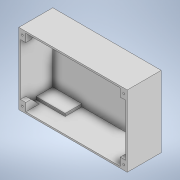
# Autodesk Inventor part: Box2
Saved by Autodesk Inventor 2022 (Build 260153000, 153)
## iProperties
Created: 2021-07-04
Part Number: Box2
Material: Generic
Document SubType Name: Modeling
Designer: Matthijs
Density: 1 g/cm^3
Appearance: Default
Author: Matthijs
Autodesk Inventor part; units mm, degrees
ref_plane "YZ Plane" through (0, 0, 0) normal (1, 0, 0) x (0, 1, 0)
ref_plane "XZ Plane" through (0, 0, 0) normal (0, 1, 0) x (-1, 0, 0)
ref_plane "XY Plane" through (0, 0, 0) normal (0, 0, 1) x (1, 0, 0)
sketch "Sketch7" plane through (0, 0, 0) normal (0, 0, 1) x (1, 0, 0)
  line L0 (100.625, -66.125) -> (-100.625, -66.125)
  line L1 (-100.625, -66.125) -> (-100.625, 66.125)
  line L2 (-100.625, 66.125) -> (100.625, 66.125)
  line L3 (100.625, 66.125) -> (100.625, -66.125)
  line L4 (100.625, -66.125) -> (-100.625, 66.125) construction
  line L5 (-100.625, -66.125) -> (100.625, 66.125) construction
  point P0 (0, 0)
  dimension "d15" = 201.25
  dimension "d16" = 132.25
  constraints: 12 end point, 2 midpoint, 2 parallel, 1 horizontal, 1 perpendicular
  measures "d15" distance of L1.end L2.end
  measures "d16" distance of L0.end L1.end
extrude "Box Outside" add sketch "Sketch7" along normal blind 63
sketch "Sketch8" plane through (0, 0, 63) normal (0, 0, 1) x (1, 0, 0)
  line L0 (-97.625, 63.125) -> (97.625, 63.125)
  line L1 (97.625, 63.125) -> (97.625, -63.125)
  line L2 (97.625, -63.125) -> (-97.625, -63.125)
  line L3 (-97.625, -63.125) -> (-97.625, 63.125)
  line L4 (100.625, 66.125) -> (-100.625, 66.125) projected
  line L5 (-100.625, 66.125) -> (-100.625, -66.125) projected
  line L6 (-100.625, -66.125) -> (100.625, -66.125) projected
  line L7 (100.625, -66.125) -> (100.625, 66.125) projected
  point P0 (0, 0)
  dimension "d19" = 3
  dimension "d20" = 3
  dimension "d21" = 3
  dimension "d22" = 3
  constraints: 8 end point, 2 parallel, 1 horizontal, 1 perpendicular
  measures "d19" distance between parallel lines of L4 L0
  measures "d20" distance between parallel lines of L5 L3
  measures "d21" distance between parallel lines of L6 L2
  measures "d22" distance between parallel lines of L7 L1
extrude "Box Cut" cut sketch "Sketch8" against normal blind 60 contours L0 L1 L2 L3
sketch "Sketch9" plane through (-97.625, -63.125, 63) normal (0, 1, 0) x (1, 0, 0)
  line L0 (0, 0) -> (10, 0)
  line L1 (10, 0) -> (10, 25)
  line L2 (10, 25) -> (0, 25)
  line L3 (0, 25) -> (0, 0)
  point P0 (97.625, 63)
  dimension "d25" = 10
  dimension "d26" = 25
  constraints: 8 end point, 2 parallel, 1 horizontal, 1 perpendicular
  measures "d25" distance of L2.end L1.end
  measures "d26" distance of L1.end L0.end
extrude "ScrewHole Box LB" add sketch "Sketch9" along normal blind 15
sketch "Sketch10" plane through (-97.625, -63.125, 3) normal (0, 1, 0) x (1, 0, 0)
  line L0 (195.25, -60) -> (195.25, 0) projected
  line L1 (195.25, -60) -> (185.25, -60)
  line L2 (185.25, -60) -> (185.25, -35)
  line L3 (185.25, -35) -> (195.25, -35)
  line L4 (195.25, -35) -> (195.25, -60)
  point P0 (97.625, 3)
  dimension "d29" = 10
  dimension "d30" = 25
  constraints: 8 end point, 2 parallel, 1 horizontal, 1 perpendicular
  measures "d29" distance of L2.end L3.end
  measures "d30" distance of L1.end L2.end
extrude "ScrewHole Box RB" add sketch "Sketch10" along normal blind 15
sketch "Sketch11" plane through (-97.625, 63.125, 63) normal (0, -1, 0) x (1, 0, 0)
  line L0 (0, 0) -> (195.25, 0) projected
  line L1 (0, 0) -> (10, 0)
  line L2 (10, 0) -> (10, -25)
  line L3 (10, -25) -> (0, -25)
  line L4 (0, -25) -> (0, 0)
  point P0 (97.625, -63)
  dimension "d33" = 10
  dimension "d34" = 25
  constraints: 8 end point, 2 parallel, 1 horizontal, 1 perpendicular
  measures "d33" distance of L2.end L3.end
  measures "d34" distance of L1.end L2.end
extrude "ScrewHole Box LU" add sketch "Sketch11" along normal blind 15
sketch "Sketch13" plane through (97.625, -63.125, 3) normal (-1, 0, 0) x (0, 0, 1)
  line L0 (60, 126.25) -> (0, 126.25) projected
  line L1 (60, 126.25) -> (35, 126.25)
  line L2 (35, 126.25) -> (35, 111.25)
  line L3 (35, 111.25) -> (60, 111.25)
  line L4 (60, 111.25) -> (60, 126.25)
  point P0 (-3, 63.125)
  dimension "d37" = 25
  dimension "d38" = 15
  constraints: 8 end point, 2 parallel, 1 horizontal, 1 perpendicular
  measures "d37" distance of L3.end L2.end
  measures "d38" distance of L2.end L1.end
extrude "ScrewHole Box RU" add sketch "Sketch13" along normal blind 10
sketch "Sketch27" plane through (0, 0, 63) normal (0, 0, 1) x (1, 0, 0)
  line L0 (-87.625, -63.125) -> (-87.625, -48.125) projected
  line L1 (-100.625, 66.125) -> (-100.625, -66.125) projected
  line L2 (-87.625, -48.125) -> (-100.625, -48.125)
  line L3 (-100.625, -48.125) -> (-100.625, -66.125)
  line L4 (-100.625, -66.125) -> (-87.625, -66.125)
  line L5 (-87.625, -66.125) -> (-87.625, -48.125)
  line L6 (-87.625, -48.125) -> (-100.625, -66.125)
  line L7 (-87.625, -66.125) -> (-100.625, -48.125)
  circle A0 centre (-94.125, -57.125) radius 2.4
  point P0 (0, 0)
  dimension "d84" = 4.8
  constraints: 12 end point, 2 parallel, 1 centre point, 1 coincident, 1 horizontal, 1 midpoint, 1 perpendicular
  measures "d84" diameter of A0
extrude "Outside ScrewHole LB" cut sketch "Sketch27" against normal blind 26 contours A0 L7 L6 | L6 L7 A0 | A0 L6 L7 | L7 L6 A0
sketch "Sketch29" plane through (0, 0, 63) normal (0, 0, 1) x (1, 0, 0)
  line L0 (-87.625, -63.125) -> (-87.625, -48.125) projected
  line L1 (-100.625, -66.125) -> (100.625, -66.125) projected
  line L2 (-87.625, -48.125) -> (-100.625, -48.125)
  line L3 (-100.625, -48.125) -> (-100.625, -66.125)
  line L4 (-100.625, -66.125) -> (-87.625, -66.125)
  line L5 (-87.625, -66.125) -> (-87.625, -48.125)
  line L6 (-87.625, -48.125) -> (-100.625, -66.125)
  circle A0 centre (-94.125, -57.125) radius 2.4
  point P0 (0, 0)
  constraints: 10 end point, 2 parallel, 1 centre point, 1 coincident, 1 horizontal, 1 midpoint, 1 perpendicular
extrude "ScrewRibbon LB" add sketch "Sketch29" against normal blind 2 contours A0 L6 | L6 A0
sketch "Sketch30" plane through (0, 0, 63) normal (0, 0, 1) x (1, 0, 0)
  line L0 (-97.625, -48.125) -> (-87.625, -48.125) projected
  line L1 (-100.625, -66.125) -> (100.625, -66.125) projected
  line L2 (-87.625, -48.125) -> (-100.625, -48.125)
  line L3 (-100.625, -48.125) -> (-100.625, -66.125)
  line L4 (-100.625, -66.125) -> (-87.625, -66.125)
  line L5 (-87.625, -66.125) -> (-87.625, -48.125)
  line L6 (-87.625, -48.125) -> (-100.625, -66.125)
  circle A0 centre (-94.125, -57.125) radius 1.7
  point P0 (0, 0)
  dimension "d92" = 3.4
  constraints: 10 end point, 2 parallel, 1 centre point, 1 coincident, 1 horizontal, 1 midpoint, 1 perpendicular
  measures "d92" diameter of A0
extrude "Inside ScrewHole LB" cut sketch "Sketch30" against normal blind 24 contours A0 L6 | L6 A0
sketch "Sketch31" plane through (0, 0, 63) normal (0, 0, 1) x (1, 0, 0)
  line L0 (-100.625, 66.125) -> (-100.625, -66.125) projected
  line L1 (-87.625, 48.125) -> (-97.625, 48.125) projected
  line L2 (-100.625, 66.125) -> (-87.625, 66.125)
  line L3 (-87.625, 66.125) -> (-87.625, 48.125)
  line L4 (-87.625, 48.125) -> (-100.625, 48.125)
  line L5 (-100.625, 48.125) -> (-100.625, 66.125)
  line L6 (-100.625, 66.125) -> (-87.625, 48.125)
  circle A0 centre (-94.125, 57.125) radius 2.4
  point P0 (0, 0)
  dimension "d95" = 4.8
  constraints: 10 end point, 2 parallel, 1 centre point, 1 coincident, 1 horizontal, 1 midpoint, 1 perpendicular
  measures "d95" diameter of A0
extrude "Outside ScrewHole LU" cut sketch "Sketch31" against normal blind 24 contours A0 L6 | L6 A0
sketch "Sketch32" plane through (0, 0, 63) normal (0, 0, 1) x (1, 0, 0)
  line L0 (-97.625, 48.125) -> (-87.625, 48.125) projected
  line L1 (-100.625, 66.125) -> (-100.625, -66.125) projected
  line L2 (-87.625, 48.125) -> (-100.625, 48.125)
  line L3 (-100.625, 48.125) -> (-100.625, 66.125)
  line L4 (-100.625, 66.125) -> (-87.625, 66.125)
  line L5 (-87.625, 66.125) -> (-87.625, 48.125)
  line L6 (-87.625, 66.125) -> (-100.625, 48.125)
  circle A0 centre (-94.125, 57.125) radius 2.4
  point P0 (0, 0)
  dimension "d98" = 4.8
  constraints: 10 end point, 2 parallel, 1 centre point, 1 coincident, 1 horizontal, 1 midpoint, 1 perpendicular
  measures "d98" diameter of A0
extrude "ScrewRibbon LU" add sketch "Sketch32" against normal blind 2 contours A0 L6 | L6 A0
sketch "Sketch33" plane through (0, 0, 63) normal (0, 0, 1) x (1, 0, 0)
  line L0 (100.625, 66.125) -> (-100.625, 66.125) projected
  line L1 (-87.625, 48.125) -> (-97.625, 48.125) projected
  line L2 (-100.625, 66.125) -> (-87.625, 66.125)
  line L3 (-87.625, 66.125) -> (-87.625, 48.125)
  line L4 (-87.625, 48.125) -> (-100.625, 48.125)
  line L5 (-100.625, 48.125) -> (-100.625, 66.125)
  line L6 (-100.625, 66.125) -> (-87.625, 48.125)
  circle A0 centre (-94.125, 57.125) radius 1.7
  point P0 (0, 0)
  dimension "d101" = 3.4
  constraints: 10 end point, 2 parallel, 1 centre point, 1 coincident, 1 horizontal, 1 midpoint, 1 perpendicular
  measures "d101" diameter of A0
extrude "Inside ScrewHole LU" cut sketch "Sketch33" against normal blind 21.75 contours A0 L6 | L6 A0
sketch "Sketch34" plane through (0, 0, 63) normal (0, 0, 1) x (1, 0, 0)
  line L0 (87.625, 48.125) -> (87.625, 63.125) projected
  line L1 (100.625, 66.125) -> (-100.625, 66.125) projected
  line L2 (87.625, 48.125) -> (100.625, 48.125)
  line L3 (100.625, 48.125) -> (100.625, 66.125)
  line L4 (100.625, 66.125) -> (87.625, 66.125)
  line L5 (87.625, 66.125) -> (87.625, 48.125)
  line L6 (100.625, 66.125) -> (87.625, 48.125)
  circle A0 centre (94.125, 57.125) radius 2.4
  point P0 (0, 0)
  dimension "d104" = 4.8
  constraints: 10 end point, 2 parallel, 1 centre point, 1 coincident, 1 horizontal, 1 midpoint, 1 perpendicular
  measures "d104" diameter of A0
extrude "Outside ScrewHole RU" cut sketch "Sketch34" against normal blind 37 contours A0 L6 | L6 A0
sketch "Sketch35" plane through (0, 0, 63) normal (0, 0, 1) x (1, 0, 0)
  line L0 (100.625, -66.125) -> (100.625, 66.125) projected
  line L1 (97.625, 48.125) -> (87.625, 48.125) projected
  line L2 (100.625, 66.125) -> (87.625, 66.125)
  line L3 (87.625, 66.125) -> (87.625, 48.125)
  line L4 (87.625, 48.125) -> (100.625, 48.125)
  line L5 (100.625, 48.125) -> (100.625, 66.125)
  line L6 (100.625, 66.125) -> (-100.625, 66.125) projected
  line L7 (100.625, 66.125) -> (87.625, 48.125)
  circle A0 centre (94.125, 57.125) radius 2.4
  point P0 (0, 0)
  dimension "d107" = 4.8
  constraints: 10 end point, 2 parallel, 1 centre point, 1 coincident, 1 horizontal, 1 midpoint, 1 perpendicular
  measures "d107" diameter of A0
extrude "ScrewRibbon RU" add sketch "Sketch35" against normal blind 2 contours A0 L7 | L7 A0
sketch "Sketch36" plane through (0, 0, 63) normal (0, 0, 1) x (1, 0, 0)
  line L0 (97.625, 48.125) -> (87.625, 48.125) projected
  line L1 (100.625, -66.125) -> (100.625, 66.125) projected
  line L2 (87.625, 48.125) -> (100.625, 48.125)
  line L3 (100.625, 48.125) -> (100.625, 66.125)
  line L4 (100.625, 66.125) -> (87.625, 66.125)
  line L5 (87.625, 66.125) -> (87.625, 48.125)
  line L6 (87.625, 48.125) -> (100.625, 66.125)
  circle A0 centre (94.125, 57.125) radius 2.4 projected
  circle A1 centre (94.125, 57.125) radius 1.7
  point P0 (0, 0)
  dimension "d110" = 3.4
  constraints: 10 end point, 2 coincident, 2 parallel, 1 centre point, 1 horizontal, 1 perpendicular
  measures "d110" diameter of A1
extrude "Inside ScrewHole RU" cut sketch "Sketch36" against normal blind 20 contours A1 L6 | L6 A1
sketch "Sketch37" plane through (0, 0, 63) normal (0, 0, 1) x (1, 0, 0)
  line L0 (100.625, -66.125) -> (100.625, 66.125) projected
  line L1 (87.625, -63.125) -> (87.625, -48.125) projected
  line L2 (100.625, -66.125) -> (87.625, -66.125)
  line L3 (87.625, -66.125) -> (87.625, -48.125)
  line L4 (87.625, -48.125) -> (100.625, -48.125)
  line L5 (100.625, -48.125) -> (100.625, -66.125)
  line L6 (87.625, -66.125) -> (100.625, -48.125)
  circle A0 centre (94.125, -57.125) radius 2.4
  point P0 (0, 0)
  dimension "d113" = 4.8
  constraints: 10 end point, 2 parallel, 1 centre point, 1 coincident, 1 horizontal, 1 midpoint, 1 perpendicular
  measures "d113" diameter of A0
extrude "Outside ScrewHole RB" cut sketch "Sketch37" against normal blind 27.5 contours A0 L6 | L6 A0
sketch "Sketch38" plane through (0, 0, 63) normal (0, 0, 1) x (1, 0, 0)
  line L0 (97.625, -48.125) -> (87.625, -48.125) projected
  line L1 (100.625, -66.125) -> (100.625, 66.125) projected
  line L2 (87.625, -48.125) -> (100.625, -48.125)
  line L3 (100.625, -48.125) -> (100.625, -66.125)
  line L4 (100.625, -66.125) -> (87.625, -66.125)
  line L5 (87.625, -66.125) -> (87.625, -48.125)
  line L6 (100.625, -48.125) -> (87.625, -66.125)
  circle A0 centre (94.125, -57.125) radius 2.4
  point P0 (0, 0)
  dimension "d116" = 4.8
  constraints: 10 end point, 2 parallel, 1 centre point, 1 coincident, 1 horizontal, 1 midpoint, 1 perpendicular
  measures "d116" diameter of A0
extrude "ScrewRibbon RB" add sketch "Sketch38" against normal blind 2 contours A0 L6 | L6 A0
sketch "Sketch39" plane through (0, 0, 63) normal (0, 0, 1) x (1, 0, 0)
  line L0 (87.625, -63.125) -> (87.625, -48.125) projected
  line L1 (100.625, -66.125) -> (100.625, 66.125) projected
  line L2 (87.625, -48.125) -> (100.625, -48.125)
  line L3 (100.625, -48.125) -> (100.625, -66.125)
  line L4 (100.625, -66.125) -> (87.625, -66.125)
  line L5 (87.625, -66.125) -> (87.625, -48.125)
  line L6 (87.625, -66.125) -> (100.625, -48.125)
  circle A0 centre (94.125, -57.125) radius 2.4 projected
  circle A1 centre (94.125, -57.125) radius 1.7
  point P0 (0, 0)
  dimension "d119" = 3.4
  constraints: 10 end point, 2 coincident, 2 parallel, 1 centre point, 1 horizontal, 1 perpendicular
  measures "d119" diameter of A1
extrude "Inside ScrewHole RB" cut sketch "Sketch39" against normal blind 20 contours A1 L6 | L6 A1
sketch "Sketch42" plane through (-97.625, -63.125, 3) normal (0, 1, 0) x (1, 0, 0)
  line L0 (195.25, 0) -> (0, 0) projected
  line L1 (0, 0) -> (54, 0)
  line L2 (54, 0) -> (54, -31)
  line L3 (54, -31) -> (0, -31)
  line L4 (0, -31) -> (0, 0)
  line L5 (0, -35) -> (0, 0) projected
  point P0 (97.625, 3)
  point P1 (54, 0)
  dimension "d134" = 54
  dimension "d135" = 31
  dimension "d167" = 0
  constraints: 8 end point, 2 parallel, 1 horizontal, 1 perpendicular, 1 point on line
  measures "d134" distance of L2.end L3.end
  measures "d135" distance of L1.end L2.end
  measures "d167" distance between parallel lines of L5 L4
extrude "ESPHolder" add sketch "Sketch42" along normal blind 5
chamfer "Chamfer1" distance 15 angle 45 1 edges at (-92.625, -48.125, 38)
chamfer "Chamfer2" distance 15 angle 45 1 edges at (-92.625, 48.125, 38)
chamfer "Chamfer3" distance 15 angle 45 1 edges at (92.625, 48.125, 38)
chamfer "Chamfer4" distance 15 angle 45 1 edges at (92.625, -48.125, 38)
body "Solid2"
